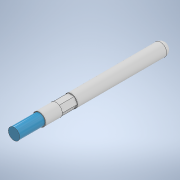
# Autodesk Inventor part: Thermoelement
Saved by Autodesk Inventor 2021 (Build 250183000, 183)
## iProperties
Created: 2021-05-06
Part Number: Thermoelement
Material: Generisch
Document SubType Name: Modeling
Designer: Sebastian Seewald
Density: 1 g/cm^3
Appearance: Vorgabe
Author: Sebastian Seewald
Autodesk Inventor part; units mm, degrees
ref_plane "YZ Plane" through (0, 0, 0) normal (1, 0, 0) x (0, 1, 0)
ref_plane "XY Plane" through (0, 0, 0) normal (0, 0, 1) x (1, 0, 0)
sketch "Skizze1" plane through (0, 0, 0) normal (0, 0, 1) x (1, 0, 0)
  circle A0 centre (0, 0) radius 2.5
  dimension "d0" = 5
  constraints: 1 centre point, 1 coincident
  measures "d0" diameter of A0
extrude "Extrusion1" add sketch "Skizze1" along normal blind 50
fillet "Rundung1" radius 2.2 1 edges at (-2.5, 0, 0)
ref_plane "Arbeitsebene1" through (0, 2.5, 0) normal (0, 1, 0) x (-1, 0, 0)
sketch "Skizze2" plane through (0, 2.5, 0) normal (0, 1, 0) x (-1, 0, 0)
  line L0 (2.5, 2.2) -> (2.5, 50) projected
  line L1 (-2.5, 2.2) -> (-2.5, 50) projected
  line L2 (2.5, 43.4257) -> (-2.5, 43.4257)
  line L3 (-2.5, 43.4257) -> (-2.5, 37.4257)
  line L4 (-2.5, 37.4257) -> (2.5, 37.4257)
  line L5 (2.5, 37.4257) -> (2.5, 43.4257)
  point P0 (0, 0)
  point P1 (-2.5, 43.4257)
  dimension "d4" = 6
  constraints: 8 end point, 2 parallel, 2 point on line, 1 horizontal, 1 perpendicular
  measures "d4" distance between parallel lines of L2 L4
extrude "Extrusion2" cut sketch "Skizze2" against normal blind 0.4
pattern_circular "Runde Anordnung1" count 6 over 360 about axis through (0, 0, -10) along (0, 0, 1) of "Extrusion2"
sketch "Skizze3" plane through (0, 0, 50) normal (0, 0, 1) x (1, 0, 0)
  circle A0 centre (0, 0) radius 2.25
  dimension "d10" = 4.5
  constraints: 1 centre point, 1 coincident
  measures "d10" diameter of A0
extrude "Extrusion3" add sketch "Skizze3" along normal blind 10
